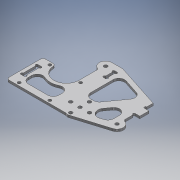
# Autodesk Inventor part: 付け根_メインフレーム_2_1
Saved by Autodesk Inventor 2018 (Build 220112000, 112)
## iProperties
Created: 2018-10-11
Part Number: 付け根_メインフレーム_2_1
Material: アルミニウム 2014-T4
Document SubType Name: Modeling
Designer: taka
Density: 2.8 g/cm^3
Appearance: サテン
d38: 10.000 mm
d39: 0.025 mm
d40: 2.100 mm
d41: 0.025 mm
Author: taka
Autodesk Inventor part; units mm, degrees
ref_plane "YZ Plane" through (0, 0, 0) normal (1, 0, 0) x (0, 1, 0)
ref_plane "XZ Plane" through (0, 0, 0) normal (0, 1, 0) x (-1, 0, 0)
ref_plane "XY Plane" through (0, 0, 0) normal (0, 0, 1) x (1, 0, 0)
derived "付け根_メイン基準フレーム.ipt"
sketch "スケッチ1" plane through (0, 0, 0) normal (0, 0, 1) x (1, 0, 0)
  circle A0 centre (32, -20) radius 4.05
  line L0 (21.5, 30) -> (61, 30) construction
  line L1 (61, 30) -> (61, -21.5) construction
  line L2 (61, -21.5) -> (21.5, -21.5) construction
  line L3 (21.5, -21.5) -> (21.5, 30) construction
  line L4 (21.5, 18) -> (61, 18) construction
  line L5 (16, 28.5) -> (66.5, 28.5) construction
  line L6 (66.5, 28.5) -> (66.5, 7.5) construction
  line L7 (66.5, 7.5) -> (16, 7.5) construction
  line L8 (16, 7.5) -> (16, 28.5) construction
  line L9 (-13.5, -1) -> (13.5, -1) construction
  line L10 (13.5, -1) -> (13.5, -28) construction
  line L11 (13.5, -28) -> (-13.5, -28) construction
  line L12 (-13.5, -28) -> (-13.5, -1) construction
  circle A1 centre (-13.5, -1) radius 1.35
  circle A2 centre (13.5, -1) radius 1.35
  circle A3 centre (-13.5, -28) radius 1.35
  circle A4 centre (13.5, -28) radius 1.35
  line L13 (10.583, 12) -> (-10.583, 12) construction
  line L14 (16, -0.88) -> (16, -39.5) construction
  line L15 (16, -39.5) -> (-16, -39.5) construction
  line L16 (-16, -39.5) -> (-16, 0) construction
  arc A5 (16, -0.88) -> (10.583, 12) centre (-2.0208, -0.88) ccw construction
  arc A6 (-10.583, 12) -> (-16, 0) centre (0, 0) ccw construction
  line L17 (35.05, -18.2391) -> (35.05, -21.7609) construction
  line L18 (35.05, -21.7609) -> (32, -23.5218) construction
  line L19 (32, -23.5218) -> (28.95, -21.7609) construction
  line L20 (28.95, -21.7609) -> (28.95, -18.2391) construction
  line L21 (28.95, -18.2391) -> (32, -16.4782) construction
  line L22 (32, -16.4782) -> (35.05, -18.2391) construction
  line L23 (0, 12) -> (0, 0) construction
  line L24 (0, 0) -> (0, -1) construction
  circle A7 centre (0, 0) radius 10.5 construction
  point P0 (0, 0)
  point P1 (66.5, 18)
sketch "スケッチ3" plane through (0, 0, 0) normal (0, 0, 1) x (1, 0, 0)
  circle A0 centre (61, -16.5) radius 5.5 construction
  line L0 (61, -21.5) -> (21.5, -21.5) construction
  line L1 (61, 30) -> (61, -21.5) construction
  line L2 (64.05, -18.2609) -> (61, -20.0218) construction
  line L3 (61, -20.0218) -> (57.95, -18.2609) construction
  line L4 (57.95, -18.2609) -> (57.95, -14.7391) construction
  line L5 (57.95, -14.7391) -> (61, -12.9782) construction
  line L6 (61, -12.9782) -> (64.05, -14.7391) construction
  line L7 (64.05, -14.7391) -> (64.05, -18.2609) construction
  circle A1 centre (32, -20) radius 1.55
  circle A2 centre (32, -20) radius 5.5 construction
  circle A3 centre (32, -11.75) radius 2.75 construction
  circle A4 centre (32, -11.75) radius 1.55
  circle A5 centre (23.75, -20) radius 1.55
  circle A6 centre (32, -28.25) radius 1.55
  circle A7 centre (40.25, -20) radius 1.55
  line L8 (-16, -39.5) -> (-16, 0) construction
  circle A8 centre (-13.5, -28) radius 2.5 construction
  circle A9 centre (-13.5, -1) radius 2.5 construction
  circle A10 centre (13.5, -1) radius 2.5 construction
  circle A11 centre (13.5, -28) radius 2.5 construction
  line L9 (-16, -30.5) -> (-22, -30.5)
  line L10 (-22, -30.5) -> (-22, 1.5)
  line L11 (-22, 1.5) -> (-11.037, 1.5)
  line L12 (-16, -6) -> (-19, -6) construction
  line L13 (-19, -6) -> (-19, -21) construction
  line L14 (-19, -21) -> (-16, -21) construction
  line L15 (-16, -21) -> (-16, -6) construction
  line L16 (-19.025, -5.975) -> (-15.975, -5.975)
  line L17 (-15.975, -5.975) -> (-15.975, -21.025)
  line L18 (-15.975, -21.025) -> (-19.025, -21.025)
  line L19 (-19.025, -21.025) -> (-19.025, -5.975)
  line L20 (-19.025, -13.5) -> (-15.975, -13.5) construction
  line L21 (-17.5, -5.975) -> (-17.5, -21.025) construction
  circle A12 centre (-19.025, -7.025) radius 1.05
  circle A13 centre (-19.025, -19.975) radius 1.05
  circle A14 centre (-15.975, -7.025) radius 1.05
  circle A15 centre (-15.975, -19.975) radius 1.05
  line L22 (61, 7.5) -> (65, 7.5)
  line L23 (65, -0.5) -> (61, -0.5)
  arc A16 (61, 9.6) -> (61, 7.5) centre (61, 8.55) ccw
  arc A17 (61, -0.5) -> (61, -2.6) centre (61, -1.55) ccw
  line L24 (65, 7.5) -> (65, -0.5)
  line L25 (61, 9.6) -> (61, 7.5) construction
  line L26 (61, 15.2) -> (61, 9.6)
  circle A18 centre (13, 22.5) radius 5.5 construction
  line L27 (16.05, 20.7391) -> (13, 18.9782) construction
  line L28 (13, 18.9782) -> (9.95, 20.7391) construction
  line L29 (9.95, 20.7391) -> (9.95, 24.2609) construction
  line L30 (9.95, 24.2609) -> (13, 26.0218) construction
  line L31 (13, 26.0218) -> (16.05, 24.2609) construction
  line L32 (16.05, 24.2609) -> (16.05, 20.7391) construction
  line L33 (16, 7.5) -> (16, 28.5) construction
  line L34 (21.5, 18) -> (61, 18) construction
  line L35 (16, 28) -> (13, 28)
  circle A19 centre (32, -28.25) radius 2.75 construction
  circle A20 centre (-13.5, -1) radius 1.35 projected
  circle A21 centre (13.5, -1) radius 1.35 projected
  circle A22 centre (13.5, -28) radius 1.35 projected
  circle A23 centre (-13.5, -28) radius 1.35 projected
  arc A24 (-11.037, 0) -> (11.037, 0) centre (0, 0) ccw
  line L36 (-11.037, 1.5) -> (-11.037, 0)
  line L37 (-16, 0) -> (15.9774, 0) construction
  line L38 (11.037, 0) -> (11.037, 17.3622)
  arc A25 (13, 28) -> (11.037, 17.3622) centre (13, 22.5) ccw
  line L39 (61, -2.6) -> (61, -11)
  line L40 (19.5, 23) -> (21.5, 23) construction
  line L41 (21.5, 23) -> (21.5, 13) construction
  line L42 (21.5, 13) -> (19.5, 13) construction
  line L43 (19.5, 13) -> (19.5, 23) construction
  line L44 (21.525, 23.025) -> (19.475, 23.025) construction
  line L45 (19.475, 23.025) -> (19.475, 12.975) construction
  line L46 (19.475, 12.975) -> (21.525, 12.975) construction
  line L47 (21.525, 12.975) -> (21.525, 23.025) construction
  circle A26 centre (19.475, 21.975) radius 1.05 construction
  arc A27 (19.475, 23.025) -> (19.475, 20.925) centre (19.475, 21.975) ccw
  line L48 (20.5, 12.975) -> (20.5, 23.025) construction
  line L49 (19.5, 18) -> (21.5, 18) construction
  line L50 (19.475, 23.025) -> (21.525, 23.025)
  arc A28 (21.525, 20.925) -> (21.525, 23.025) centre (21.525, 21.975) ccw
  line L51 (21.525, 20.925) -> (21.525, 15.075)
  line L52 (19.475, 20.925) -> (19.475, 15.075)
  arc A29 (19.475, 15.075) -> (19.475, 12.975) centre (19.475, 14.025) ccw
  line L53 (19.475, 12.975) -> (21.525, 12.975)
  arc A30 (21.525, 12.975) -> (21.525, 15.075) centre (21.525, 14.025) ccw
  line L54 (21.5, -21.5) -> (21.5, 30) construction
  circle A31 centre (61, -16.5) radius 1.55
  circle A32 centre (13, 22.5) radius 1.55
  line L55 (21.5, 28) -> (61, 15.2)
  line L56 (16, 28) -> (21.5, 28)
  line L57 (16, 28.5) -> (66.5, 28.5) construction
  line L58 (32, -20) -> (32, -11.75) construction
  line L59 (-16, -30.5) -> (30.4189, -30.5)
  line L60 (32.8047, -30.8796) -> (62.6094, -21.7593)
  arc A33 (62.6094, -21.7593) -> (61, -11) centre (61, -16.5) ccw
  arc A34 (30.4189, -30.5) -> (32.8047, -30.8796) centre (32, -28.25) ccw
  dimension "d40" = 2.1
  dimension "d3" = 11
  dimension "d4" = 6.1
  dimension "d5" = 3.1
  dimension "d6" = 11
  dimension "d7" = 5.5
  dimension "d8" = 3.1
  dimension "d11" = 360
  dimension "d13" = 6
  dimension "d14" = 3
  dimension "d15" = 15
  dimension "d16" = 0.025
  dimension "d17" = 2.1
  dimension "d22" = 2.1
  dimension "d23" = 1.05
  dimension "d24" = 2.1
  dimension "d25" = 1.05
  dimension "d26" = 8
  dimension "d27" = 4
  dimension "d31" = 11
  dimension "d32" = 6.1
  dimension "d35" = 5.5
  dimension "d38" = 10
  dimension "d39" = 0.025
  dimension "d42" = 2
  dimension "d45" = 3.1
  dimension "d46" = 3.1
  dimension "d75" = 7.7
  dimension "d82" = 15
  dimension "d84" = 5
  dimension "d86" = 21
  dimension "d87" = 0.5
  dimension "d91" = 3
  constraints: 108 end point, 30 centre point, 26 point on circle, 16 coincident, 11 parallel, 11 tangent, 8 horizontal, 8 perpendicular, 8 vertical, 7 equal radius, 7 midpoint, 7 point on line, 7 symmetric about line, 6 collinear, 1 concentric, 1 line through centre, 1 vertical alignment, 55 other
  measures "d3" diameter of A0
  measures "d4" distance between parallel lines of L7 L4
  measures "d5" diameter of A1
  measures "d6" diameter of A2
  measures "d7" diameter of A3
  measures "d8" diameter of A4
  measures "d13" distance of L9.start L9.end
  measures "d14" distance of L14.end L14.start
  measures "d15" distance of L14.start L13.start
  measures "d16" distance between parallel lines of L12 L16
  measures "d17" diameter of A12
  measures "d22" distance of L22.start L25.start
  measures "d23" radius of A16
  measures "d24" distance of L23.end L39.start
  measures "d25" radius of A17
  measures "d26" distance between parallel lines of L23 L22
  measures "d27" distance of L22.end L22.start
  measures "d31" diameter of A18
  measures "d32" distance between parallel lines of L32 L29
  measures "d35" diameter of A19
  measures "d38" distance of L42.end L40.start
  measures "d39" distance between parallel lines of L44 L40
  measures "d42" distance between parallel lines of L54 L43
  measures "d45" diameter of A31
  measures "d46" diameter of A32
  measures "d75" distance from line of L22 L26.start
  measures "d82" distance between parallel lines of L20 L11
  measures "d84" distance from line of L0 A31.centre
  measures "d86" distance between parallel lines of L22 L57
  measures "d87" distance between parallel lines of L56 L57
  measures "d91" distance from line of L33 A18.centre
extrude "押し出し3" add sketch "スケッチ3" along normal blind 2
sketch "スケッチ5" plane through (0, 0, 0) normal (0, 0, -1) x (-1, 0, 0)
  circle A0 centre (-13, 22.5) radius 1.55 projected
  circle A1 centre (-61, -16.5) radius 1.55 projected
  line L0 (-58.2, -18.1166) -> (-61, -19.7332)
  line L1 (-61, -19.7332) -> (-63.8, -18.1166)
  line L2 (-63.8, -18.1166) -> (-63.8, -14.8834)
  line L3 (-63.8, -14.8834) -> (-61, -13.2668)
  line L4 (-61, -13.2668) -> (-58.2, -14.8834)
  line L5 (-58.2, -14.8834) -> (-58.2, -18.1166)
  line L6 (-11.3834, 25.3) -> (-9.7668, 22.5)
  line L7 (-9.7668, 22.5) -> (-11.3834, 19.7)
  line L8 (-11.3834, 19.7) -> (-14.6166, 19.7)
  line L9 (-14.6166, 19.7) -> (-16.2332, 22.5)
  line L10 (-16.2332, 22.5) -> (-14.6166, 25.3)
  line L11 (-14.6166, 25.3) -> (-11.3834, 25.3)
  circle A2 centre (-61, -14.3168) radius 1.05
  line L12 (-61, 30) -> (-61, -21.5) construction
  circle A3 centre (-62.8907, -15.4084) radius 1.05
  circle A4 centre (-62.8907, -17.5916) radius 1.05
  circle A5 centre (-61, -18.6832) radius 1.05
  circle A6 centre (-59.1093, -17.5916) radius 1.05
  circle A7 centre (-59.1093, -15.4084) radius 1.05
  circle A8 centre (-15.1832, 22.5) radius 1.05
  line L13 (-16.2332, 22.5) -> (-13, 22.5) construction
  circle A9 centre (-14.0916, 20.6093) radius 1.05
  circle A10 centre (-11.9084, 20.6093) radius 1.05
  circle A11 centre (-10.8168, 22.5) radius 1.05
  circle A12 centre (-11.9084, 24.3907) radius 1.05
  circle A13 centre (-14.0916, 24.3907) radius 1.05
  point P0 (0, 0)
  point P1 (-63.8, -14.8834)
  point P2 (-63.8, -18.1166)
  point P3 (-61, -19.7332)
  point P4 (-58.2, -18.1166)
  point P5 (-58.2, -14.8834)
  point P6 (-14.6166, 19.7)
  point P7 (-11.3834, 19.7)
  point P8 (-9.7668, 22.5)
  dimension "d50" = 2.1
  dimension "d56" = 2.1
  dimension "d49" = 5.6
  dimension "d53" = 360
  dimension "d55" = 5.6
  dimension "d59" = 360
  constraints: 26 end point, 2 coincident, 2 horizontal alignment, 2 vertical, 2 vertical alignment, 1 horizontal, 1 point on line, 96 other
  measures "d49" distance between parallel lines of L5 L2
  measures "d55" distance between parallel lines of L11 L8
extrude "押し出し4" cut sketch "スケッチ5" against normal blind 0.25 contours A0 A11 | A0 A11 L6 L7 | A0 A12 L6 A11 | A11 L7 A10 A0 | A12 A0 | A0 A12 L11 L6 | A11 L6 | A10 L7 L8 A0 | A0 A10 | L7 A11 | A0 A13 L11 A12 | L6 A12 | A10 L8 A9 A0 | A10 L7 | A13 A0 | A0 A13 L10 L11 | A12 L11 | A9 L8 L9 A0 | A0 A9 | L8 A10 | A0 A8 L10 A13 | L11 A13 | A9 L9 A8 A0 | A9 L8 | A8 A0 | A0 A8 L9 L10 | A13 L10 | L9 A9 | L10 A8 | A8 L9 | A1 A7 L5 A6 | A7 A1 | A1 A7 L4 L5 | A6 L5 L0 A1 | A1 A6 | A1 A2 L4 A7 | L5 A7 | A6 L0 A5 A1 | A6 L5 | A2 A1 | A1 A2 L3 L4 | A7 L4 | A5 L0 L1 A1 | A1 A5 | L0 A6 | A1 A3 L3 A2 | L4 A2 | A5 L1 A4 A1 | A5 L0 | A3 A1 | A1 A3 L2 L3 | A2 L3 | A4 L1 L2 A1 | A1 A4 | L1 A5 | A1 A4 L2 A3 | L3 A3 | A4 L1 | A3 L2 | L2 A4
sketch "スケッチ6" plane through (0, 0, 2) normal (0, 0, 1) x (1, 0, 0)
  circle A0 centre (32, -20) radius 1.55 projected
  circle A1 centre (32, -11.75) radius 1.55 projected
  circle A2 centre (32, -11.75) radius 2.75 construction
  circle A3 centre (32, -20) radius 11 construction
  circle A4 centre (-13.5, -28) radius 1.35 projected
  circle A5 centre (13.5, -28) radius 1.35 projected
  circle A6 centre (13.5, -1) radius 1.35 projected
  circle A7 centre (-13.5, -1) radius 1.35 projected
  circle A8 centre (-13.5, -1) radius 3 construction
  circle A9 centre (-13.5, -28) radius 3 construction
  circle A10 centre (13.5, -28) radius 3 construction
  circle A11 centre (13.5, -1) radius 3 construction
  arc A12 (13, 28) -> (11.037, 17.3622) centre (13, 22.5) ccw projected
  circle A13 centre (13, 22.5) radius 5.5 construction
  arc A14 (55.6162, -17.6246) -> (55.5, -16.5) centre (61, -16.5) ccw construction
  line L0 (-13.5, -4) -> (-13.5, -25)
  line L1 (-13.5, -28) -> (-13.5, -1) construction
  arc A15 (-13.5, -4) -> (13.5, -4) centre (0, 0) ccw
  line L2 (13.5, -4) -> (13.5, -25)
  line L3 (-13.5, -25) -> (13.5, -25)
  line L4 (25.5, -11.1259) -> (25.5, 12.0709)
  line L5 (21.5, -21.5) -> (21.5, 30) construction
  line L6 (61, 9.6) -> (61, 15.2) projected
  line L7 (25.5, -11.1259) -> (25.5, -21.5174) construction
  line L8 (25.5, -21.5174) -> (42.8948, -21.5174) construction
  line L9 (25.5, 22.499) -> (25.5, 22.499) construction
  line L10 (55.5, 12.7775) -> (55.5, 6.7707) construction
  line L11 (42.8948, -21.5174) -> (53.6527, -18.2254)
  line L12 (52.0053, 13.91) -> (41.7671, -0.3701)
  line L13 (40.9208, -13.5642) -> (44.8744, -8.0497)
  line L14 (25.5, 22.499) -> (52.0053, 13.91)
  line L15 (25.5, 12.0709) -> (25.5, 22.499)
  line L16 (52.0053, 13.91) -> (55.5, 12.7775) construction
  line L17 (55.5, 6.7707) -> (55.5, -15.0245)
  line L18 (41.7671, -0.3701) -> (39.4243, -3.638)
  line L19 (39.4243, -3.638) -> (35.2318, -9.4855)
  line L20 (47.2173, -4.7819) -> (55.5, 6.7707)
  line L21 (44.8744, -8.0497) -> (47.2173, -4.7819)
  line L22 (55.5, -15.0245) -> (55.5, -16.5)
  line L23 (53.6527, -18.2254) -> (55.6162, -17.6246)
  arc A16 (35.2318, -9.4855) -> (25.5, -11.1259) centre (32, -20) ccw
  arc A17 (42.8948, -21.5174) -> (40.9208, -13.5642) centre (32, -20) ccw
  line L24 (61, 15.2) -> (21.5, 28) projected
  line L25 (25.5, 22.499) -> (25.5, 18.0219)
  arc A18 (55.5, -16.5) -> (55.6162, -17.6246) centre (61, -16.5) ccw
  line L26 (55.5, 12.7775) -> (32, -20) construction
  arc A19 (62.6094, -21.7593) -> (61, -11) centre (61, -16.5) ccw projected
  line L27 (32.8047, -30.8796) -> (62.6094, -21.7593) projected
  point P0 (21.5, 27)
  point P1 (21.5, 28)
  point P2 (21.525, 20.925)
  dimension "d64" = 6
  dimension "d63" = 5.5
  dimension "d66" = 4
  dimension "d74" = 7
  dimension "d80" = 4
  dimension "d89" = 5.5
  dimension "d90" = 6
  constraints: 46 end point, 14 point on circle, 10 coincident, 10 parallel, 8 centre point, 6 vertical, 4 perpendicular, 4 point on line, 4 vertical alignment, 3 collinear, 2 concentric, 2 horizontal, 2 tangent, 12 other
  measures "d63" diameter of A2
  measures "d66" distance between parallel lines of L4 L5
  measures "d74" distance between parallel lines of L13 L12
  measures "d89" distance between parallel lines of L6 L17
  measures "d90" distance between parallel lines of L27 L11
extrude "押し出し5" cut sketch "スケッチ6" against normal through all contours A15 L2 L3 L0 | L4 L15 L14 L12 L18 L19 A16 | A17 L13 L21 L20 L17 L22 A18 L23 L11
fillet "フィレット1" radius 5 12 edges at (13.5, -4, 1) (-13.5, -4, 1) (-13.5, -25, 1) (13.5, -25, 1) (25.5, -11.1259, 1) (35.2318, -9.4855, 1) (25.5, 22.499, 1) (52.0053, 13.91, 1) (55.5, 6.7707, 1) (42.8948, -21.5174, 1) (40.9208, -13.5642, 1) (55.6162, -17.6246, 1)
fillet "フィレット1" radius 2 4 edges at (11.037, 17.3622, 1) (61, -11, 1) (-11.037, 1.5, 1) (30.4189, -30.5, 1)
chamfer "面取り1" distance 5.5 angle 45 2 edges at (-22, 1.5, 1) (-22, -30.5, 1)
fillet "フィレット2" radius 2 4 edges at (-16.5, 1.5, 1) (-22, -4, 1) (-22, -25, 1) (-16.5, -30.5, 1)
equation "\"d22\" = 2 * d23"
equation "\"d24\" = d22"
equation "\"d25\" = d23"
